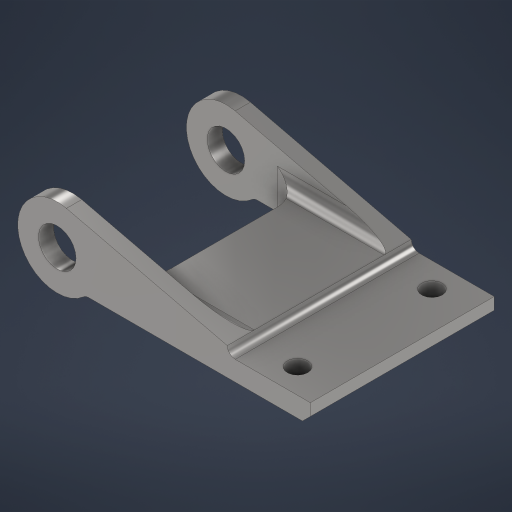
# Autodesk Inventor part: Part2
Saved by Autodesk Inventor 2023 (Build 270158000, 158)
## iProperties
Created: 2022-11-27
Part Number: Part2
Material: Stainless Steel
Document SubType Name: Modeling
Designer: iusti
Density: 8 g/cm^3
Appearance: Semi-Polished
Author: iusti
Autodesk Inventor part; units mm, degrees
ref_plane "YZ Plane" through (0, 0, 0) normal (1, 0, 0) x (0, 1, 0)
ref_plane "XZ Plane" through (0, 0, 0) normal (0, 1, 0) x (-1, 0, 0)
ref_plane "XY Plane" through (0, 0, 0) normal (0, 0, 1) x (1, 0, 0)
sketch "Sketch1" plane through (0, 0, 0) normal (0, 0, 1) x (1, 0, 0)
  arc A0 (2.3256, 9.7258) -> (7.1414, -7) centre (0, 0) ccw
  line L0 (7.1414, -7) -> (64, -7)
  line L1 (64, -7) -> (64, -2)
  line L2 (64, -2) -> (45, -2)
  arc A1 (43, 0) -> (45, -2) centre (45, 0) ccw
  line L3 (43, 0) -> (2.3256, 9.7258)
  dimension "d0" = 20
  dimension "d1" = 21
  dimension "d2" = 64
  dimension "d3" = 5
  dimension "d4" = 2
  dimension "d5" = 7
  constraints: 8 end point, 4 point on circle, 2 centre point, 2 perpendicular, 2 tangent, 1 coincident, 1 horizontal, 1 horizontal alignment
  measures "d0" diameter of A0
  measures "d1" distance from line of L3.start L1
  measures "d2" distance from line of L1 point (0, 0)
  measures "d3" distance of L0.end L1.end
  measures "d4" radius of A1
  measures "d5" distance from line of L0 point (0, 0)
extrude "Extrusion1" add sketch "Sketch1" along normal mid plane 46.5
sketch "Sketch2" plane through (0, 0, 23.25) normal (0, 0, 1) x (1, 0, 0)
  arc A0 (2.3256, 9.7258) -> (7.1414, -7) centre (0, 0) ccw projected
  constraints: 1 coincident
hole "Hole1" at (0, 0, 23.25) direction (0, 0, -1) diameter 9.5 depth 46.5
sketch "Sketch4" plane through (64, -7, 23.25) normal (1, 0, 0) x (0, 0, -1)
  line L0 (46.5, 17) -> (0, 17) projected
  line L1 (46.5, 7) -> (0, 7) projected
  line L2 (3.85, 17) -> (42.65, 17)
  line L3 (42.65, 17) -> (42.65, 10)
  line L4 (39.65, 7) -> (6.85, 7)
  line L5 (3.85, 10) -> (3.85, 17)
  arc A0 (3.85, 10) -> (6.85, 7) centre (6.85, 10) ccw
  arc A1 (39.65, 7) -> (42.65, 10) centre (39.65, 10) ccw
  point P0 (23.25, 7)
  point P1 (23.25, 7)
  dimension "d20" = 38.8
  dimension "d21" = 3
  constraints: 8 end point, 4 point on circle, 4 tangent, 2 centre point, 2 midpoint, 2 parallel, 1 collinear, 1 equal radius, 1 horizontal, 1 perpendicular
  measures "d20" distance of L2.start L2.end
  measures "d21" radius of A0
extrude "Extrusion3" cut sketch "Sketch4" against normal up to next
sketch "Sketch6" plane through (0, 0, 0) normal (0, 1, 0) x (-1, 0, 0)
  line L0 (10, 16.4) -> (10, -16.4) projected
  line L1 (-2.3256, -19.4) -> (-30.4537, -19.4) projected
  line L2 (-30.4537, 19.4) -> (-2.3256, 19.4) projected
  line L3 (10, -19.4) -> (-13, -19.4)
  line L4 (-19, -13.4) -> (-19, 13.4)
  line L5 (-13, 19.4) -> (10, 19.4)
  line L6 (10, 19.4) -> (10, -19.4)
  arc A0 (-19, -13.4) -> (-13, -19.4) centre (-13, -13.4) ccw
  arc A1 (-13, 19.4) -> (-19, 13.4) centre (-13, 13.4) ccw
  point P0 (0, 0)
  point P1 (-19, -19.4)
  point P2 (10, 0)
  point P3 (-13, -19.4)
  point P4 (-2.3256, 19.4)
  point P5 (-13, 19.4)
  dimension "d24" = 38.8
  dimension "d26" = 6
  dimension "d29" = 19
  constraints: 8 end point, 4 point on circle, 4 tangent, 2 centre point, 2 midpoint, 2 parallel, 2 point on line, 1 equal radius, 1 horizontal, 1 perpendicular
  measures "d24" distance of L5.end L3.start
  measures "d26" radius of A0
  measures "d29" distance from line of L4 point (0, 0)
extrude "Extrusion4" cut sketch "Sketch6" along normal through all both and the other way through all
sketch "Sketch7" plane through (45, -2, 23.25) normal (0, 1, 0) x (1, 0, 0)
  line L0 (19, 46.5) -> (19, 0) projected
  line L1 (9.5, 40.25) -> (9.5, 6.25) construction
  line L2 (19, 46.5) -> (19, 0) construction
  point P0 (-45, 23.25)
  point P1 (9.5, 23.25)
  dimension "d31" = 34
  dimension "d33" = 9.5
  constraints: 2 end point, 1 horizontal alignment, 1 midpoint, 1 vertical
  measures "d31" distance of L1.start L1.end
  measures "d33" distance between parallel lines of L0 L1
hole "Hole2" at (54.5, -2, 17) at (54.5, -2, -17) direction (0, -1, 0) diameter 5.2 end through all
chamfer "Chamfer1" distance 2 angle 45 1 edges at (64, -7, 0)
fillet "Fillet1" radius 2 2 edges at (7.1414, -7, 21.325) (7.1414, -7, -21.325)
body "Solid1"
